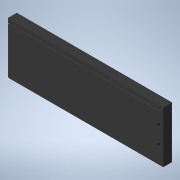
# Autodesk Inventor part: CubeBase_in
Saved by Autodesk Inventor 2020 (Build 240168000, 168)
## iProperties
Created: 2019-12-01
Part Number: CubeBase_in
Material: Generic
Document SubType Name: Modeling
Designer: torto
Density: 1 g/cm^3
Appearance: Default
Author: torto
Autodesk Inventor part; units mm, degrees
ref_plane "YZ Plane" through (0, 0, 0) normal (1, 0, 0) x (0, 1, 0)
ref_plane "XZ Plane" through (0, 0, 0) normal (0, 1, 0) x (-1, 0, 0)
ref_plane "XY Plane" through (0, 0, 0) normal (0, 0, 1) x (1, 0, 0)
sketch "Sketch1" plane through (0, 0, 0) normal (0, 0, 1) x (1, 0, 0)
  line L0 (0, 0) -> (228.6, 0)
  line L1 (228.6, 0) -> (228.6, 76.2)
  line L2 (228.6, 76.2) -> (0, 76.2)
  line L3 (0, 76.2) -> (0, 0)
  line L4 (228.6, 76.2) -> (222.25, 76.2) construction
  line L5 (222.25, 76.2) -> (222.25, 69.85) construction
  line L6 (222.25, 69.85) -> (228.6, 69.85) construction
  line L7 (228.6, 69.85) -> (228.6, 76.2) construction
  line L8 (222.25, 69.85) -> (0, 69.85)
  line L9 (0, 69.85) -> (0, 68.326)
  line L10 (0, 68.326) -> (222.25, 68.326)
  line L11 (222.25, 68.326) -> (222.25, 69.85)
  line L12 (228.6, 0) -> (222.25, 0) construction
  line L13 (222.25, 0) -> (222.25, 25.4) construction
  line L14 (222.25, 25.4) -> (228.6, 25.4) construction
  line L15 (228.6, 25.4) -> (228.6, 0) construction
  circle A0 centre (222.25, 25.4) radius 2.5146
  circle A1 centre (222.25, 50.8) radius 2.5146
  dimension "d0" = 228.6
  dimension "height" = 76.2
  dimension "d3" = 6.35
  dimension "d4" = 6.35
  dimension "d5" = 222.25
  dimension "d6" = 1.524
  dimension "spacing" = 25.4
  dimension "d9" = 6.35
  dimension "d10" = 5.0292
  dimension "d13" = 25.4
  constraints: 32 end point, 8 parallel, 4 horizontal, 4 perpendicular, 2 centre point, 2 coincident, 1 vertical, 3 other
  measures "d0" distance of L2.end L1.end
  measures "height" distance of L1.end L0.end
  measures "d3" distance of L5.end L4.end
  measures "d4" distance of L5.end L6.end
  measures "d5" distance of L10.end L9.end
  measures "d6" distance of L9.end L8.end
  measures "spacing" distance of L12.end L13.end
  measures "d9" distance of L13.end L14.end
  measures "d10" diameter of A0
  measures "d13" distance of A0.centre A1.centre
extrude "Generic Shape" add sketch "Sketch1" along normal blind 12.7
sketch "Sketch2" plane through (0, 0, 12.7) normal (0, 0, 1) x (1, 0, 0)
  line L0 (228.6, 76.2) -> (0, 76.2) construction
  line L1 (228.6, 76.2) -> (222.25, 76.2) construction
  line L2 (222.25, 76.2) -> (222.25, 69.85) construction
  line L3 (222.25, 69.85) -> (228.6, 69.85) construction
  line L4 (228.6, 69.85) -> (228.6, 76.2) construction
  line L5 (222.25, 69.85) -> (0, 69.85)
  line L6 (0, 69.85) -> (0, 68.326)
  line L7 (0, 68.326) -> (222.25, 68.326)
  line L8 (222.25, 68.326) -> (222.25, 69.85)
  point P0 (0, 0)
  dimension "d21" = 6.35
  dimension "d22" = 6.35
  dimension "d23" = 222.25
  dimension "d24" = 1.524
  constraints: 16 end point, 4 parallel, 2 horizontal, 2 perpendicular
  measures "d21" distance of L2.end L1.end
  measures "d22" distance of L2.end L3.end
  measures "d23" distance of L7.end L6.end
  measures "d24" distance of L6.end L5.end
extrude "PCB Notch" cut sketch "Sketch2" against normal blind 6.35
sketch "Sketch3" plane through (0, 0, 12.7) normal (0, 0, 1) x (1, 0, 0)
  point P0 (0, 0)
sketch "Sketch4" plane through (0, 0, 0) normal (-1, 0, 0) x (0, 0, 1)
  line L0 (0, 0) -> (6.35, 0) construction
  line L1 (6.35, 0) -> (6.35, 25.4) construction
  line L2 (6.35, 25.4) -> (0, 25.4) construction
  line L3 (0, 25.4) -> (0, 0) construction
  circle A0 centre (6.35, 25.4) radius 2.5146
  line L4 (0, 76.2) -> (6.35, 76.2) construction
  line L5 (6.35, 76.2) -> (6.35, 50.8) construction
  line L6 (6.35, 50.8) -> (0, 50.8) construction
  line L7 (0, 50.8) -> (0, 76.2) construction
  circle A1 centre (6.35, 50.8) radius 2.5146
  dimension "d33" = 6.35
  dimension "d34" = 25.4
  dimension "d35" = 5.0292
  dimension "d36" = 6.35
  dimension "d37" = 25.4
  dimension "d38" = 5.0292
  constraints: 16 end point, 4 parallel, 2 centre point, 2 coincident, 2 horizontal, 2 perpendicular
  measures "d33" distance of L2.end L1.end
  measures "d34" distance of L1.end L0.end
  measures "d35" diameter of A0
  measures "d36" distance of L5.end L6.end
  measures "d37" distance of L4.end L5.end
  measures "d38" diameter of A1
extrude "2in Screw Depth" cut sketch "Sketch4" against normal blind 50.8
thread "M5-0.8-2.0in (1)" size "M5x0.8" class "6H" standard "ANSI Metric M Profile" full length
thread "M5-0.8-2.0in (2)" size "M5x0.8" class "6H" standard "ANSI Metric M Profile" full length
sketch "Screw Caps" plane through (0, 0, 0) normal (0, 0, -1) x (-1, 0, 0)
  circle A0 centre (-222.25, 25.4) radius 2.5146 projected
  circle A1 centre (-222.25, 25.4) radius 4.375
  circle A2 centre (-222.25, 50.8) radius 2.5146 projected
  circle A3 centre (-222.25, 50.8) radius 4.375
  point P0 (0, 0)
  dimension "d45" = 8.75
  dimension "d46" = 8.75
  constraints: 2 centre point, 2 coincident
  measures "d45" diameter of A1
  measures "d46" diameter of A3
extrude "Screw Caps 5M-0.8" cut sketch "Screw Caps" against normal blind 5.0292 contours A0 | A1 | A2 | A3
equation "\"spacing\" = 0.333333 * height"
equation "\"d13\" = spacing"
body "Solid1"
